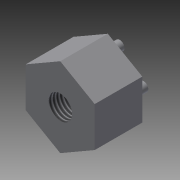
# Autodesk Inventor part: Nut
Saved by Autodesk Inventor 2015 (Build 190159000, 159)
## iProperties
Created: 2016-04-14
Part Number: Nut
Material: Generic
Document SubType Name: Modeling
Designer: Diogo Figueiredo
Density: 1 g/cm^3
Appearance: Default
Author: Diogo Figueiredo
Autodesk Inventor part; units mm, degrees
ref_plane "YZ Plane" through (0, 0, 0) normal (1, 0, 0) x (0, 1, 0)
ref_plane "XZ Plane" through (0, 0, 0) normal (0, 1, 0) x (-1, 0, 0)
ref_plane "XY Plane" through (0, 0, 0) normal (0, 0, 1) x (1, 0, 0)
sketch "Sketch1" plane through (0, 0, 0) normal (0, 1, 0) x (-1, 0, 0)
  line L0 (0, -16.7083) -> (-14.4698, -8.3542)
  line L1 (-14.4698, -8.3542) -> (-14.4698, 8.3542)
  line L2 (-14.4698, 8.3542) -> (0, 16.7083)
  line L3 (0, 16.7083) -> (14.4698, 8.3542)
  line L4 (14.4698, 8.3542) -> (14.4698, -8.3542)
  line L5 (14.4698, -8.3542) -> (0, -16.7083)
  circle A0 centre (0, 0) radius 5
  dimension "d0" = 10
  constraints: 12 end point, 2 coincident, 1 centre point, 13 other
  measures "d0" diameter of A0
extrude "Extrusion1" add sketch "Sketch1" along normal blind 20
thread "Thread1" size "M10x1.5" class "6H" standard "ANSI Metric M Profile" full length
sketch "Sketch2" plane through (0, 20, 0) normal (0, 1, 0) x (1, 0, 0)
  circle A0 centre (-10, 0) radius 2
  circle A1 centre (0, 10) radius 2
  circle A2 centre (0, -10) radius 2
  circle A3 centre (10, 0) radius 2
  point P0 (0, 0)
  dimension "d6" = 4
  dimension "d7" = 4
  dimension "d8" = 4
  dimension "d9" = 4
  constraints: 4 centre point
  measures "d6" diameter of A0
  measures "d7" diameter of A1
  measures "d8" diameter of A2
  measures "d9" diameter of A3
extrude "Extrusion2" add sketch "Sketch2" along normal blind 5
body "Solid1"
